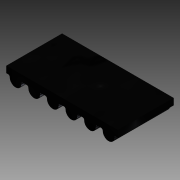
# Autodesk Inventor part: 520-5M-15
Saved by Autodesk Inventor 2013 (Build 170138000, 138)
## iProperties
Category: Drive Base Kit
Company: Autodesk Inc.
Created: 2012-12-27
Part Number: 520-5M-15
Material: Nylon 6/6
Document SubType Name: Modeling
Designer: Autodesk Inc.
Density: 1 g/cm^3
Catalog Web Link: www.andymark.inc
Vendor: AndyMark Inc.
Author: Autodesk Inc.
Autodesk Inventor part; units mm, degrees
ref_plane "YZ Plane" through (0, 0, 0) normal (1, 0, 0) x (0, 1, 0)
ref_plane "XZ Plane" through (0, 0, 0) normal (0, 1, 0) x (-1, 0, 0)
ref_plane "XY Plane" through (0, 0, 0) normal (0, 0, 1) x (1, 0, 0)
sketch "Sketch1" plane through (0, 0, 0) normal (0, 0, 1) x (1, 0, 0)
  line L0 (0.9375, -2.1467) -> (0.9375, -2.2475)
  arc A0 (0.9375, -2.2475) -> (4.0625, -2.2475) centre (2.5, -2.2475) ccw
  line L1 (4.0625, -2.2475) -> (4.0625, -2.1467)
  arc A1 (4.4792, -1.73) -> (4.0625, -2.1467) centre (4.4792, -2.1467) ccw
  line L2 (4.4792, -1.73) -> (5.5208, -1.73)
  arc A2 (5.9375, -2.1467) -> (5.5208, -1.73) centre (5.5208, -2.1467) ccw
  line L3 (5.9375, -2.1467) -> (5.9375, -2.2475)
  arc A3 (5.9375, -2.2475) -> (9.0625, -2.2475) centre (7.5, -2.2475) ccw
  line L4 (9.0625, -2.2475) -> (9.0625, -2.1467)
  arc A4 (9.4792, -1.73) -> (9.0625, -2.1467) centre (9.4792, -2.1467) ccw
  line L5 (9.4792, -1.73) -> (10.5208, -1.73)
  arc A5 (10.9375, -2.1467) -> (10.5208, -1.73) centre (10.5208, -2.1467) ccw
  line L6 (10.9375, -2.1467) -> (10.9375, -2.2475)
  arc A6 (10.9375, -2.2475) -> (14.0625, -2.2475) centre (12.5, -2.2475) ccw
  line L7 (14.0625, -2.2475) -> (14.0625, -2.1467)
  arc A7 (14.4792, -1.73) -> (14.0625, -2.1467) centre (14.4792, -2.1467) ccw
  line L8 (14.4792, -1.73) -> (15.5208, -1.73)
  arc A8 (15.9375, -2.1467) -> (15.5208, -1.73) centre (15.5208, -2.1467) ccw
  line L9 (15.9375, -2.1467) -> (15.9375, -2.2475)
  arc A9 (15.9375, -2.2475) -> (19.0625, -2.2475) centre (17.5, -2.2475) ccw
  line L10 (19.0625, -2.2475) -> (19.0625, -2.1467)
  arc A10 (19.4792, -1.73) -> (19.0625, -2.1467) centre (19.4792, -2.1467) ccw
  line L11 (19.4792, -1.73) -> (20.5208, -1.73)
  arc A11 (20.9375, -2.1467) -> (20.5208, -1.73) centre (20.5208, -2.1467) ccw
  line L12 (20.9375, -2.1467) -> (20.9375, -2.2475)
  arc A12 (20.9375, -2.2475) -> (24.0625, -2.2475) centre (22.5, -2.2475) ccw
  line L13 (24.0625, -2.2475) -> (24.0625, -2.1467)
  arc A13 (24.4792, -1.73) -> (24.0625, -2.1467) centre (24.4792, -2.1467) ccw
  line L14 (24.4792, -1.73) -> (25.5208, -1.73)
  arc A14 (25.9375, -2.1467) -> (25.5208, -1.73) centre (25.5208, -2.1467) ccw
  line L15 (25.9375, -2.1467) -> (25.9375, -2.2475)
  arc A15 (25.9375, -2.2475) -> (29.0625, -2.2475) centre (27.5, -2.2475) ccw
  line L16 (29.0625, -2.2475) -> (29.0625, -2.1467)
  arc A16 (29.4792, -1.73) -> (29.0625, -2.1467) centre (29.4792, -2.1467) ccw
  line L17 (29.4792, -1.73) -> (30, -1.73)
  line L18 (30, -1.73) -> (30, 0)
  line L19 (30, 0) -> (0, 0)
  line L20 (0, 0) -> (0, -1.73)
  line L21 (0, -1.73) -> (0.5208, -1.73)
  arc A17 (0.9375, -2.1467) -> (0.5208, -1.73) centre (0.5208, -2.1467) ccw
  point P0 (25, 0)
  constraints: 44 end point, 36 point on circle, 18 centre point
extrude "Extrusion1" add sketch "Sketch1" against normal blind 15
body "Solid1"
